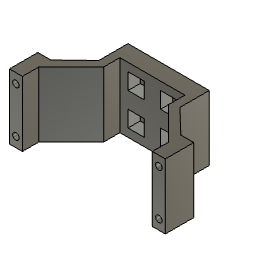
cementform_Wmiddle_80x40_plateA (Autodesk Fusion 360 design; units mm, degrees)
Autodesk Fusion 360 part; units mm, degrees
note: some values were not read from the file. Set by a fixed rule: which sketch regions a step uses.
sketch "baseplate" plane through (0, 0, 0) normal (0, 1, 0) x (1, 0, 0)
  line L0 (0, 0) -> (80, 0)
  line L1 (80, 0) -> (80, -40)
  line L2 (80, -40) -> (0, -40)
  line L3 (0, -40) -> (0, 0)
  dimension "d1" = 40
  dimension "d2" = 80
  constraint horizontal L0
  constraint vertical L1
  constraint horizontal L2
  constraint vertical L3
  constraint coincident L0.start L3.end
  measures "d1" distance of L0.start L2.end
  measures "d2" distance of L0.start L0.end
extrude "Extrude1" add sketch "baseplate" along normal blind 10
sketch "outside_pryamid" plane through (0, 0, 0) normal (0, 1, 0) x (1, 0, 0)
  line L0 (25, -35) -> (35, -35)
  line L1 (35, -35) -> (35, -25)
  line L2 (35, -25) -> (25, -25)
  line L3 (25, -25) -> (25, -35)
  line L4 (45, -35) -> (55, -35)
  line L5 (55, -35) -> (55, -25)
  line L6 (55, -25) -> (45, -25)
  line L7 (45, -25) -> (45, -35)
  line L8 (25, -15) -> (35, -15)
  line L9 (35, -15) -> (35, -5)
  line L10 (35, -5) -> (25, -5)
  line L11 (25, -5) -> (25, -15)
  line L12 (45, -15) -> (55, -15)
  line L13 (55, -15) -> (55, -5)
  line L14 (55, -5) -> (45, -5)
  line L15 (45, -5) -> (45, -15)
  constraint horizontal L0
  constraint vertical L1
  constraint horizontal L2
  constraint vertical L3
  constraint horizontal L4
  constraint vertical L5
  constraint horizontal L6
  constraint vertical L7
  constraint horizontal L8
  constraint vertical L9
  constraint horizontal L10
  constraint vertical L11
  constraint horizontal L12
  constraint vertical L13
  constraint horizontal L14
  constraint vertical L15
ref_plane "WorkPlane1" through (0, 5, 0) normal (0, 1, 0) x (0, 0, 1)
sketch "inside_pryamid" plane through (0, 5, 0) normal (0, 1, 0) x (1, 0, 0)
  line L0 (32.5, -7.5) -> (27.5, -7.5)
  line L1 (27.5, -10) -> (27.5, -12.5)
  line L2 (32.5, -12.5) -> (32.5, -7.5)
  line L3 (27.5, -7.5) -> (27.5, -10)
  line L4 (27.5, -12.5) -> (32.5, -12.5)
  line L5 (47.5, -7.5) -> (47.5, -10)
  line L6 (47.5, -12.5) -> (52.5, -12.5)
  line L7 (52.5, -7.5) -> (47.5, -7.5)
  line L8 (47.5, -10) -> (47.5, -12.5)
  line L9 (52.5, -12.5) -> (52.5, -7.5)
  line L10 (27.5, -10) -> (27.5, -12.5)
  line L11 (27.5, -12.5) -> (32.5, -12.5)
  line L12 (32.5, -12.5) -> (32.5, -7.5)
  line L13 (47.5, -7.5) -> (47.5, -10)
  line L14 (52.5, -12.5) -> (52.5, -7.5)
  line L15 (47.5, -10) -> (47.5, -12.5)
  line L16 (52.5, -7.5) -> (47.5, -7.5)
  line L17 (47.5, -12.5) -> (52.5, -12.5)
  line L18 (32.5, -7.5) -> (27.5, -7.5)
  line L19 (27.5, -7.5) -> (27.5, -10)
  line L20 (47.5, -30) -> (47.5, -32.5)
  line L21 (47.5, -32.5) -> (52.5, -32.5)
  line L22 (47.5, -32.5) -> (52.5, -32.5)
  line L23 (52.5, -32.5) -> (52.5, -27.5)
  line L24 (52.5, -27.5) -> (47.5, -27.5)
  line L25 (52.5, -27.5) -> (47.5, -27.5)
  line L26 (47.5, -30) -> (47.5, -32.5)
  line L27 (27.5, -30) -> (27.5, -32.5)
  line L28 (32.5, -27.5) -> (27.5, -27.5)
  line L29 (27.5, -32.5) -> (32.5, -32.5)
  line L30 (52.5, -32.5) -> (52.5, -27.5)
  line L31 (27.5, -27.5) -> (27.5, -30)
  line L32 (32.5, -32.5) -> (32.5, -27.5)
  line L33 (27.5, -32.5) -> (32.5, -32.5)
  line L34 (27.5, -30) -> (27.5, -32.5)
  line L35 (47.5, -27.5) -> (47.5, -30)
  line L36 (47.5, -27.5) -> (47.5, -30)
  line L37 (32.5, -32.5) -> (32.5, -27.5)
  line L38 (32.5, -27.5) -> (27.5, -27.5)
  line L39 (27.5, -27.5) -> (27.5, -30)
  constraint perpendicular L1 L4
  constraint perpendicular L2 L4
  constraint perpendicular L0 L2
  constraint perpendicular L6 L8
  constraint perpendicular L6 L9
  constraint perpendicular L7 L9
  constraint perpendicular L10 L11
  constraint perpendicular L11 L12
  constraint perpendicular L12 L18
  constraint perpendicular L15 L17
  constraint perpendicular L14 L17
  constraint perpendicular L14 L16
  constraint perpendicular L27 L33
  constraint perpendicular L32 L33
  constraint perpendicular L32 L38
  constraint perpendicular L20 L21
  constraint perpendicular L21 L30
  constraint perpendicular L25 L30
  constraint perpendicular L29 L34
  constraint perpendicular L29 L37
  constraint perpendicular L28 L37
  constraint perpendicular L22 L26
  constraint perpendicular L22 L23
  constraint perpendicular L23 L24
loft "Loft2" cut profiles "outside_pryamid", "inside_pryamid" section 1 contours L0 L1 L2 L3 section 2 contours L27 L28 L29 L31 L32 L33 L34 L37 L38 L39
loft "Loft3" cut profiles "outside_pryamid", "inside_pryamid" section 1 contours L4 L5 L6 L7 section 2 contours L20 L21 L22 L23 L24 L25 L26 L30 L35 L36
loft "Loft6" cut profiles "inside_pryamid", "outside_pryamid" section 1 contours L0 L1 L2 L3 L4 L10 L11 L12 L18 L19 section 2 contours L8 L9 L10 L11
loft "Loft7" cut profiles "inside_pryamid", "outside_pryamid" section 1 contours L5 L6 L7 L8 L9 L13 L14 L15 L16 L17 section 2 contours L12 L13 L14 L15
sketch "sidewall" plane through (0, 0, 0) normal (0, 1, 0) x (1, 0, 0)
  line L0 (0, 0) -> (-8, 0)
  line L1 (-8, 0) -> (-8, -40)
  line L2 (-8, -40) -> (0, -40)
  line L3 (0, -40) -> (0, 0)
  dimension "d12" = 8
  constraint horizontal L0
  constraint vertical L1
  constraint horizontal L2
  constraint vertical L3
  constraint coincident L0.start L3.end
  measures "d12" distance of L1.end L2.end
extrude "Extrude2" add sketch "sidewall" along normal blind -40 and the other way blind -10
sketch "sidemount" plane through (0, 0, 0) normal (0, 1, 0) x (1, 0, 0)
  line L0 (80, 0) -> (88, 0)
  line L1 (88, 0) -> (88, -40)
  line L2 (88, -40) -> (80, -40)
  line L3 (80, -40) -> (80, 0)
  constraint horizontal L0
  constraint vertical L1
  constraint horizontal L2
  constraint vertical L3
extrude "Extrude3" add sketch "sidemount" along normal blind 10
sketch "bolt holes" plane through (0, 0, 0) normal (0, 1, 0) x (1, 0, 0)
  circle A0 centre (-4, -34) radius 2
  circle A1 centre (-4, -6) radius 2
  circle A2 centre (-4, -34) radius 3.4
  circle A3 centre (-4, -6) radius 3.4
  circle A4 centre (84, -34) radius 2
  circle A5 centre (84, -6) radius 2
  dimension "d19" = 4
  dimension "d20" = 4
  dimension "d21" = 6.8
  dimension "d22" = 6.8
  dimension "d27" = 4
  dimension "d28" = 4
  constraint concentric A0 A2
  measures "d19" diameter of A0
  measures "d20" diameter of A1
  measures "d21" diameter of A2
  measures "d22" diameter of A3
  measures "d27" diameter of A4
  measures "d28" diameter of A5
extrude "Extrude4" cut sketch "bolt holes" against normal blind 50 contours A0 | A1
extrude "Extrude6" cut sketch "bolt holes" along normal through all and the other way blind 44 contours A0 | A1
extrude "Extrude7" cut sketch "bolt holes" along normal blind 10 and the other way blind -4 contours A2 | A3
sketch "W infill" plane through (0, 0, 0) normal (0, 0, 1) x (1, 0, 0)
  line L0 (0, 0) -> (0, -20)
  line L1 (0, 0) -> (20, 0)
  line L2 (60, 0) -> (80, 0)
  line L3 (80, 0) -> (80, -20)
  line L4 (88, 0) -> (88, -40)
  line L5 (80, -20) -> (80, -40)
  line L6 (80, -40) -> (88, -40)
  line L7 (0, -40) -> (0, -30)
  line L8 (20, 0) -> (20, -10)
  line L9 (20, -10) -> (0, -30)
  line L10 (60, 0) -> (60, -10)
  line L11 (60, -10) -> (80, -30)
  line L12 (20, 0) -> (0, 0)
  line L13 (0, -30) -> (0, 0)
  line L14 (80, 0) -> (88, 0)
  constraint coincident L0.start L1.start
  constraint vertical L0
  constraint perpendicular L0 L1
  constraint parallel L3 L5
  constraint perpendicular L4 L6
  constraint perpendicular L1 L8
  constraint perpendicular L2 L10
  constraint midpoint L5 L11.end
  constraint perpendicular L9 L11
  constraint perpendicular L0 L12
  constraint perpendicular L12 L13
  constraint perpendicular L4 L14
extrude "Extrude8" add sketch "W infill" along normal blind 40
extrude "Extrude5" cut sketch "bolt holes" along normal blind 40 and the other way blind 51 contours A4 | A5
sketch "cut off the extra" plane through (0, 0, 0) normal (0, 0, 1) x (1, 0, 0)
  line L0 (-8, 10) -> (-8, -22.5)
  line L1 (0, -22.5) -> (-8, -22.5)
  line L2 (-8, 10) -> (15, 10)
  line L3 (11.9645, -10.9645) -> (0, -22.5)
  line L4 (-8, 10) -> (-8, -22.5)
  line L5 (15, 0) -> (15, -7.9289)
  line L6 (11.9645, -10.9645) -> (15, -7.9289)
  line L7 (15, 0) -> (15, 10)
  line L8 (11.9645, -10.9645) -> (15, -7.9289)
  line L9 (11.9645, -10.9645) -> (0, -22.5)
  line L10 (15, 0) -> (15, -7.9289)
  line L11 (-8, 10) -> (-8, -22.5)
  line L12 (11.9645, -10.9645) -> (0, -22.5)
  line L13 (0, -22.5) -> (-8, -22.5)
  line L14 (11.9645, -10.9645) -> (15, -7.9289)
  line L15 (15, 0) -> (15, -7.9289)
  line L16 (88, -40) -> (88, 10)
  line L17 (88, 10) -> (65, 10)
  line L18 (65, 0) -> (65, 10)
  line L19 (88, -22.5) -> (80, -22.5)
  line L20 (68.0355, -10.9645) -> (65, -7.9289)
  line L21 (68.0355, -10.9645) -> (80, -22.5)
  line L22 (65, 0) -> (65, -7.9289)
  line L23 (88, -22.5) -> (88, 10)
  constraint parallel L5 L7
  constraint perpendicular L2 L7
  constraint perpendicular L1 L4
  constraint perpendicular L11 L13
  constraint coincident L16.end L17.start
extrude "Extrude9" cut sketch "cut off the extra" along normal blind 40
